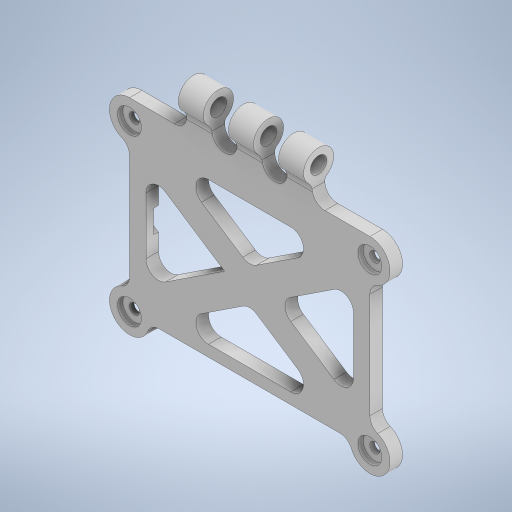
# Autodesk Inventor part: polycase_bracket
Saved by Autodesk Inventor 2024 (Build 280153000, 153)
## iProperties
Created: 2024-04-12
Part Number: polycase_bracket
Material: Generic
Document SubType Name: Modeling
Designer: Jacob
Density: 1 g/cm^3
Appearance: Default
Author: Jacob
## iProperties of the stored document polycase_bracket_3DPrint.ipt
Created: 2024-04-15
Part Number: polycase_bracket_3DPrint
Material: Generic
Document SubType Name: Modeling
Designer: Jacob
Density: 1 g/cm^3
Appearance: Default
Author: Jacob
Autodesk Inventor part; units mm, degrees
ref_plane "YZ Plane" through (0, 0, 0) normal (1, 0, 0) x (0, 1, 0)
ref_plane "XZ Plane" through (0, 0, 0) normal (0, 1, 0) x (-1, 0, 0)
ref_plane "XY Plane" through (0, 0, 0) normal (0, 0, 1) x (1, 0, 0)
sketch "Sketch1" plane through (0, 0, 0) normal (0, 0, 1) x (1, 0, 0)
  line L0 (48, -33) -> (-48, -33)
  line L1 (-48, -33) -> (-48, 33)
  line L2 (-48, 33) -> (48, 33)
  line L3 (48, 33) -> (48, -33)
  line L4 (48, -33) -> (-48, 33) construction
  line L5 (-48, -33) -> (48, 33) construction
  circle A0 centre (-48, 33) radius 1.727
  circle A1 centre (48, 33) radius 1.727
  circle A2 centre (-48, -33) radius 1.727
  circle A3 centre (48, -33) radius 1.727
  circle A4 centre (-48, 33) radius 8
  circle A5 centre (48, 33) radius 8
  circle A6 centre (48, -33) radius 8
  circle A7 centre (-48, -33) radius 8
  line L6 (41.4077, -28.4678) -> (-41.4077, -28.4678)
  line L7 (-41.4077, -28.4678) -> (-41.4077, 28.4678)
  line L8 (-41.4077, 28.4678) -> (41.4077, 28.4678)
  line L9 (41.4077, 28.4678) -> (41.4077, -28.4678)
  line L10 (41.4077, -28.4678) -> (-41.4077, 28.4678) construction
  line L11 (-41.4077, -28.4678) -> (41.4077, 28.4678) construction
  line L12 (-40, -33) -> (48, 25)
  line L13 (40, 33) -> (-48, -25)
  line L14 (-40, 33) -> (48, -25)
  line L15 (40, -33) -> (-48, 25)
  line L16 (56, 33) -> (56, -33)
  line L17 (-48, 41) -> (48, 41)
  line L18 (-56, 33) -> (-56, -33)
  line L19 (-48, -41) -> (48, -41)
  point P0 (0, 0)
  point P1 (-33.1235, -28.4678)
  point P2 (0, -6.6364)
  point P3 (33.1235, -28.4678)
  point P4 (41.4077, 20.6551)
  point P5 (41.4077, -20.6551)
  point P6 (10.069, 0)
  point P7 (33.1235, 28.4678)
  point P8 (0, 6.6364)
  point P9 (-33.1235, 28.4678)
  point P10 (-41.4077, -20.6551)
  point P11 (-41.4077, 20.6551)
  point P12 (-10.069, 0)
  dimension "d0" = 96
  dimension "d1" = 66
  dimension "d2" = 3.454
  dimension "d3" = 3.454
  dimension "d4" = 3.454
  dimension "d5" = 3.454
  dimension "d6" = 16
  dimension "d7" = 16
  dimension "d8" = 16
  dimension "d9" = 16
  constraints: 40 end point, 17 point on circle, 8 centre point, 8 coincident, 6 point on line, 4 midpoint, 4 parallel, 4 perpendicular, 2 horizontal, 2 tangent
  measures "d0" distance of L1.end L2.end
  measures "d1" distance of L0.end L1.end
  measures "d2" diameter of A0
  measures "d3" diameter of A1
  measures "d4" diameter of A2
  measures "d5" diameter of A3
  measures "d6" diameter of A4
  measures "d7" diameter of A5
  measures "d8" diameter of A6
  measures "d9" diameter of A7
extrude "Extrusion1" add sketch "Sketch1" along normal blind 5 contours A6 L3 A3 L0 | L15 L6 A6 | L0 A3 L3 A6 | L0 L12 L6 L15 | A7 L1 A2 L0 | L0 A2 L1 A7 | A7 L6 L12 | L9 L14 A6 | L6 L15 L12 L14 L9 | L7 L13 L15 L12 L6 | A7 L13 L7 | L14 L9 L12 L3 | L15 L13 L14 L12 | L1 L15 L7 L13 | A5 L2 A1 L3 | L12 L9 A5 | L3 A1 L2 A5 | L12 L14 L13 L8 L9 | L15 L7 L8 L14 L13 | A4 L2 A0 L1 | L1 A0 L2 A4 | A4 L7 L15 | L8 L13 A5 | A4 L14 L8 | L13 L8 L14 L2
fillet "Fillet1" radius 5 19 edges at (-40, 33, 2.5) (-48, 25, 2.5) (-33.1235, 28.4678, 2.5) (-41.4077, 20.6551, 2.5) (0, 6.6364, 2.5) (10.069, 0, 2.5) (33.1235, 28.4678, 2.5) (41.4077, 20.6551, 2.5) (40, 33, 2.5) (48, 25, 2.5) (41.4077, -20.6551, 2.5) (33.1235, -28.4678, 2.5) (0, -6.6364, 2.5) (-33.1235, -28.4678, 2.5) (-41.4077, -20.6551, 2.5) (48, -25, 2.5) (40, -33, 2.5) (-40, -33, 2.5) (-48, -25, 2.5)
sketch "Sketch2" plane through (0, 0, 0) normal (0, 0, -1) x (-1, 0, 0)
  circle A0 centre (-48, 33) radius 1.727 projected
  circle A1 centre (-48, 33) radius 2
  circle A2 centre (48, 33) radius 1.727 projected
  circle A3 centre (48, 33) radius 2
  circle A4 centre (48, -33) radius 1.727 projected
  circle A5 centre (48, -33) radius 2
  circle A6 centre (-48, -33) radius 1.727 projected
  circle A7 centre (-48, -33) radius 2
  circle A8 centre (-48, 33) radius 4.75
  circle A9 centre (48, 33) radius 1.727 projected
  circle A10 centre (48, 33) radius 4.75
  circle A11 centre (48, -33) radius 4.75
  circle A12 centre (-48, -33) radius 4.75
  point P0 (0, 0)
  dimension "d13" = 4
  dimension "d14" = 4
  dimension "d15" = 4
  dimension "d16" = 4
  dimension "d17" = 9.5
  dimension "d18" = 9.5
  dimension "d19" = 9.5
  dimension "d20" = 9.5
  constraints: 8 centre point, 8 coincident
  measures "d13" diameter of A1
  measures "d14" diameter of A3
  measures "d15" diameter of A5
  measures "d16" diameter of A7
  measures "d17" diameter of A8
  measures "d18" diameter of A10
  measures "d19" diameter of A11
  measures "d20" diameter of A12
extrude "Extrusion2" cut sketch "Sketch2" against normal blind 5 contours A0 | A1 | A2 | A3 | A4 | A5 | A6 | A7
extrude "Extrusion3" cut sketch "Sketch2" against normal blind 1.2 contours A8 | A10 | A11 | A12
sketch "Sketch3" plane through (-36, 33, 0) normal (0, 1, 0) x (1, 0, 0)
  line L0 (86, -5) -> (82, -5) projected
  line L1 (-14, 5) -> (86, 5)
  line L2 (86, 5) -> (86, -5)
  line L3 (86, -5) -> (-14, -5)
  line L4 (-14, -5) -> (-14, 5)
  line L5 (-14, 5) -> (86, -5) construction
  line L6 (86, 5) -> (-14, -5) construction
  line L7 (76.6154, 0) -> (92, 0) projected
  line L8 (-14, -5) -> (86, -5)
  line L9 (86, -5) -> (86, 0)
  line L10 (86, 0) -> (-14, 0)
  line L11 (-14, 0) -> (-14, -5)
  line L12 (-4.6154, -5) -> (0, -5) projected
  line L13 (76.6154, 0) -> (-4.6154, 0)
  line L14 (-4.6154, 0) -> (-4.6154, -5)
  line L15 (-4.6154, -5) -> (76.6154, -5)
  line L16 (76.6154, -5) -> (76.6154, 0)
  line L17 (11, 5) -> (61, 5)
  line L18 (61, 5) -> (61, -5)
  line L19 (61, -5) -> (11, -5)
  line L20 (11, -5) -> (11, 5)
  line L21 (11, 5) -> (61, -5) construction
  line L22 (61, 5) -> (11, -5) construction
  line L23 (0, 0) -> (72, 0) projected
  line L24 (61, -5) -> (11, -5)
  line L25 (11, -5) -> (11, 0)
  line L26 (11, 0) -> (61, 0)
  line L27 (61, 0) -> (61, -5)
  line L28 (11, -5) -> (21, -5)
  line L29 (21, -5) -> (21, 0)
  line L30 (21, 0) -> (11, 0)
  line L31 (11, 0) -> (11, -5)
  line L32 (61, -5) -> (51, -5)
  line L33 (51, -5) -> (51, 0)
  line L34 (51, 0) -> (61, 0)
  line L35 (61, 0) -> (61, -5)
  line L36 (31, 5) -> (41, 5)
  line L37 (41, 5) -> (41, -5)
  line L38 (41, -5) -> (31, -5)
  line L39 (31, -5) -> (31, 5)
  line L40 (31, 5) -> (41, -5) construction
  line L41 (41, 5) -> (31, -5) construction
  line L42 (31, 0) -> (41, 0)
  point P0 (36, 0)
  point P1 (87.0769, 0)
  dimension "d25" = 50
  dimension "d26" = 10
  dimension "d27" = 10
  dimension "d28" = 10
  constraints: 78 end point, 16 parallel, 10 midpoint, 8 horizontal, 8 perpendicular, 6 point on line
  measures "d25" distance of L18.end L19.end
  measures "d26" distance of L30.end L29.end
  measures "d27" distance of L33.end L34.end
  measures "d28" distance of L37.end L38.end
extrude "Extrusion4" add sketch "Sketch3" along normal blind 20 contours L3 L33 L10 L18 | L3 L39 L10 L37 | L3 L20 L10 L29
sketch "Sketch4" plane through (25, 33, 5) normal (1, 0, 0) x (0, 0, -1)
  line L0 (5, 0) -> (5, 20) projected
  line L1 (5, 10) -> (0, 10)
  line L2 (0, 0) -> (0, 20) projected
  line L3 (0, 20) -> (5, 20) projected
  line L4 (2.5, 20) -> (2.5, 15)
  circle A0 centre (2.5, 15) radius 3.25
  circle A1 centre (2.5, 15) radius 6
  point P0 (5, -33)
  point P1 (5, 9.5456)
  point P2 (0, 9.5456)
  point P3 (0, 12.9233)
  point P4 (0, 17.0767)
  point P5 (5, 17.0767)
  point P6 (5, 12.9233)
  dimension "d31" = 5
  dimension "d32" = 6.5
  dimension "d33" = 12
  constraints: 4 end point, 3 midpoint, 2 centre point, 2 coincident, 1 vertical
  measures "d31" distance of L4.start L4.end
  measures "d32" diameter of A0
  measures "d33" diameter of A1
extrude "Extrusion5" add sketch "Sketch4" against normal up to surface (10 mm away) contours L0 A0 L3 L2 A1
extrude "Extrusion6" cut sketch "Sketch4" against normal blind 10 contours A0 L2 L0 | L0 A0 | A0 L2
sketch "Sketch5" plane through (5, 33, 5) normal (1, 0, 0) x (0, 0, -1)
  circle A0 centre (2.5, 15) radius 3.25 projected
  arc A1 (5, 9.5456) -> (0, 9.5456) centre (2.5, 15) ccw projected
  circle A2 centre (2.5, 15) radius 6
  point P0 (5, -33)
  point P1 (0, 9.5456)
  point P2 (5, 9.5456)
  constraints: 1 centre point, 1 coincident, 1 concentric
extrude "Extrusion7" add sketch "Sketch5" against normal up to surface (10 mm away)
extrude "Extrusion8" cut sketch "Sketch5" against normal blind 10 contours A0
sketch "Sketch6" plane through (-15, 33, 5) normal (1, 0, 0) x (0, 0, -1)
  circle A0 centre (2.5, 15) radius 3.25 projected
  circle A1 centre (2.5, 15) radius 3.25
  circle A2 centre (2.5, 15) radius 6
  point P0 (5, -33)
  constraints: 2 centre point, 2 coincident
extrude "Extrusion9" add sketch "Sketch6" against normal up to surface (10 mm away)
extrude "Extrusion10" cut sketch "Sketch6" against normal up to surface (10 mm away) contours A0
fillet "Fillet2" radius 2 3 edges at (20, 42.5456, 0) (0, 42.5456, 0) (-20, 42.5456, 0)
fillet "Fillet3" radius 5 9 edges at (-20, 42.5456, 5) (0, 42.5456, 5) (20, 42.5456, 5) (15, 33, 2.5) (5, 33, 2.5) (-5, 33, 2.5) (-15, 33, 2.5) (25, 33, 2.5) (-25, 33, 2.5)
sketch "Sketch8" plane through (0, 0, 5) normal (0, 0, 1) x (1, 0, 0)
  circle A0 centre (-48, 33) radius 2 projected
  circle A1 centre (-48, 33) radius 4.75
  circle A2 centre (48, 33) radius 2 projected
  circle A3 centre (48, 33) radius 4.75
  circle A4 centre (48, -33) radius 2 projected
  circle A5 centre (48, -33) radius 4.75
  circle A6 centre (-48, -33) radius 2 projected
  circle A7 centre (-48, -33) radius 4.75
  point P0 (0, 0)
  dimension "d50" = 9.5
  dimension "d51" = 9.5
  dimension "d52" = 9.5
  dimension "d53" = 9.5
  constraints: 4 centre point, 4 coincident
  measures "d50" diameter of A1
  measures "d51" diameter of A3
  measures "d52" diameter of A5
  measures "d53" diameter of A7
extrude "Extrusion12" cut sketch "Sketch8" against normal blind 2 contours A0 | A1 | A2 | A3 | A4 | A5 | A6 | A7
sketch "Sketch9" plane through (0, 0, 0) normal (0, 0, -1) x (-1, 0, 0)
  line L0 (55.3401, -40.9684) -> (-55.3401, -40.9684) projected
  spline S0 degree 3 poles (-55.3401, -40.9684) (-55.4056, -40.9684) (-55.471, -40.9554) (-55.5315, -40.9303) (-55.5919, -40.9053) (-55.6474, -40.8682) (-55.6937, -40.822) (-55.7399, -40.7757) (-55.777, -40.7202) (-55.802, -40.6598) (-55.8271, -40.5993) (-55.8401, -40.5339) (-55.8401, -40.4684) knots 5.497939 5.497939 5.497939 5.497939 5.890562 5.890562 5.890562 6.283185 6.283185 6.283185 6.675808 6.675808 6.675808 7.068431 7.068431 7.068431 7.068431 projected
  line L1 (-55.8401, -40.4684) -> (-55.8401, 40.4684) projected
  spline S1 degree 3 poles (-55.8401, 40.4684) (-55.8401, 40.5339) (-55.8271, 40.5993) (-55.802, 40.6598) (-55.777, 40.7202) (-55.7399, 40.7757) (-55.6937, 40.822) (-55.6474, 40.8682) (-55.5919, 40.9053) (-55.5315, 40.9303) (-55.471, 40.9554) (-55.4056, 40.9684) (-55.3401, 40.9684) knots 5.497939 5.497939 5.497939 5.497939 5.890562 5.890562 5.890562 6.283185 6.283185 6.283185 6.675808 6.675808 6.675808 7.068431 7.068431 7.068431 7.068431 projected
  line L2 (-55.3401, 40.9684) -> (55.3401, 40.9684) projected
  spline S2 degree 3 poles (55.3401, 40.9684) (55.4056, 40.9684) (55.471, 40.9554) (55.5315, 40.9303) (55.5919, 40.9053) (55.6474, 40.8682) (55.6937, 40.822) (55.7399, 40.7757) (55.777, 40.7202) (55.802, 40.6598) (55.8271, 40.5993) (55.8401, 40.5339) (55.8401, 40.4684) knots 5.497939 5.497939 5.497939 5.497939 5.890562 5.890562 5.890562 6.283185 6.283185 6.283185 6.675808 6.675808 6.675808 7.068431 7.068431 7.068431 7.068431 projected
  line L3 (55.8401, 40.4684) -> (55.8401, -40.4684) projected
  spline S3 degree 3 poles (55.8401, -40.4684) (55.8401, -40.5339) (55.8271, -40.5993) (55.802, -40.6598) (55.777, -40.7202) (55.7399, -40.7757) (55.6937, -40.822) (55.6474, -40.8682) (55.5919, -40.9053) (55.5315, -40.9303) (55.471, -40.9554) (55.4056, -40.9684) (55.3401, -40.9684) knots 5.497939 5.497939 5.497939 5.497939 5.890562 5.890562 5.890562 6.283185 6.283185 6.283185 6.675808 6.675808 6.675808 7.068431 7.068431 7.068431 7.068431 projected
  line L4 (29.8976, -1.9965) -> (31.7769, -2.8744) projected
  line L5 (29.8976, -2.0069) -> (29.8976, -1.9965) projected
  line L6 (28.292, -2.9083) -> (29.8976, -2.0069) projected
  line L7 (28.292, -3.3844) -> (28.292, -2.9083) projected
  line L8 (29.8556, -2.4469) -> (28.292, -3.3844) projected
  line L9 (31.7769, -3.3844) -> (29.8556, -2.4469) projected
  line L10 (31.7769, -2.8744) -> (31.7769, -3.3844) projected
  line L11 (31.7769, 5.9658) -> (31.7769, 4.5059) projected
  line L12 (28.292, 5.9658) -> (31.7769, 5.9658) projected
  line L13 (28.292, 4.553) -> (28.292, 5.9658) projected
  line L14 (28.6687, 4.553) -> (28.292, 4.553) projected
  line L15 (28.6687, 5.542) -> (28.6687, 4.553) projected
  line L16 (29.799, 5.542) -> (28.6687, 5.542) projected
  line L17 (29.799, 4.6001) -> (29.799, 5.542) projected
  line L18 (30.1757, 4.6001) -> (29.799, 4.6001) projected
  line L19 (30.1757, 5.542) -> (30.1757, 4.6001) projected
  line L20 (31.4001, 5.542) -> (30.1757, 5.542) projected
  line L21 (31.4001, 4.5059) -> (31.4001, 5.542) projected
  line L22 (31.7769, 4.5059) -> (31.4001, 4.5059) projected
  line L23 (31.7769, 1.5391) -> (28.8115, 1.5391) projected
  line L24 (31.7769, 1.9629) -> (31.7769, 1.5391) projected
  line L25 (28.292, 1.9629) -> (31.7769, 1.9629) projected
  line L26 (28.292, 1.269) -> (28.292, 1.9629) projected
  line L27 (31.2846, 0.503) -> (28.292, 1.269) projected
  line L28 (28.292, 0.503) -> (31.2846, 0.503) projected
  line L29 (28.292, 0.0792) -> (28.292, 0.503) projected
  line L30 (31.7769, 0.0792) -> (28.292, 0.0792) projected
  line L31 (31.7769, 0.7797) -> (31.7769, 0.0792) projected
  line L32 (28.8115, 1.5391) -> (31.7769, 0.7797) projected
  line L33 (31.7769, -8.3976) -> (31.7769, -9.8574) projected
  line L34 (28.292, -8.3976) -> (31.7769, -8.3976) projected
  line L35 (28.292, -9.8104) -> (28.292, -8.3976) projected
  line L36 (28.6687, -9.8104) -> (28.292, -9.8104) projected
  line L37 (28.6687, -8.8214) -> (28.6687, -9.8104) projected
  line L38 (29.799, -8.8214) -> (28.6687, -8.8214) projected
  line L39 (29.799, -9.7633) -> (29.799, -8.8214) projected
  line L40 (30.1757, -9.7633) -> (29.799, -9.7633) projected
  line L41 (30.1757, -8.8214) -> (30.1757, -9.7633) projected
  line L42 (31.4001, -8.8214) -> (30.1757, -8.8214) projected
  line L43 (31.4001, -9.8574) -> (31.4001, -8.8214) projected
  line L44 (31.7769, -9.8574) -> (31.4001, -9.8574) projected
  line L45 (31.7769, -10.2342) -> (31.7769, -10.6536) projected
  line L46 (28.292, -10.9553) -> (31.7769, -10.2342) projected
  line L47 (28.292, -11.5204) -> (28.292, -10.9553) projected
  line L48 (31.7769, -12.2415) -> (28.292, -11.5204) projected
  line L49 (31.7769, -11.7838) -> (31.7769, -12.2415) projected
  line L50 (30.9763, -11.6367) -> (31.7769, -11.7838) projected
  line L51 (30.9763, -10.803) -> (30.9763, -11.6367) projected
  line L52 (31.7769, -10.6536) -> (30.9763, -10.803) projected
  circle A0 centre (39.4888, 19.5371) radius 4.127 projected
  line L53 (31.7769, -6.1371) -> (31.7769, -6.5609) projected
  line L54 (28.292, -6.1371) -> (31.7769, -6.1371) projected
  line L55 (28.292, -7.1231) -> (28.292, -6.1371) projected
  spline S4 degree 3 poles (29.1536, -7.8795) (29.0848, -7.8799) (28.985, -7.874) (28.8571, -7.8556) (28.772, -7.8348) (28.6936, -7.8094) (28.6229, -7.7765) (28.5583, -7.7396) (28.5018, -7.6954) (28.4517, -7.6458) (28.4091, -7.5893) (28.3725, -7.5269) (28.3436, -7.4579) (28.3194, -7.3833) (28.2983, -7.2712) (28.2908, -7.1835) (28.292, -7.1231) knots 0 0 0 0 0.156529 0.227063 0.293634 0.355378 0.41429 0.470549 0.524222 0.577081 0.630415 0.684665 0.741142 0.800246 0.862827 1 1 1 1 projected
  spline S5 degree 3 poles (29.8026, -7.6676) (29.7671, -7.7045) (29.7032, -7.7511) (29.6071, -7.7992) (29.5249, -7.8284) (29.4354, -7.8521) (29.3373, -7.8676) (29.2426, -7.877) (29.1804, -7.8793) (29.1536, -7.8795) knots 0.046127 0.046127 0.046127 0.046127 0.254948 0.367127 0.484568 0.611118 0.745389 0.890554 1 1 1 1 projected
  spline S6 degree 3 poles (29.991, -7.2614) (29.9755, -7.3413) (29.9387, -7.4908) (29.8517, -7.6179) (29.8026, -7.6676) knots 0 0 0 0 0.539837 1 1 1 1 projected
  spline S7 degree 3 poles (30.1404, -7.6588) (30.1182, -7.6394) (30.0896, -7.6041) (30.0588, -7.5498) (30.0383, -7.5028) (30.0216, -7.4499) (30.0022, -7.3696) (29.995, -7.3055) (29.991, -7.2614) knots 0 0 0 0 0.202398 0.311642 0.429962 0.556371 0.693993 1 1 1 1 projected
  spline S8 degree 3 poles (30.729, -7.7971) (30.6623, -7.7954) (30.5661, -7.7923) (30.4447, -7.7752) (30.3661, -7.7616) (30.2971, -7.7412) (30.2194, -7.7131) (30.1687, -7.6826) (30.1404, -7.6588) knots 0 0 0 0 0.326051 0.468546 0.597628 0.71466 0.819562 1 1 1 1 projected
  spline S9 degree 3 poles (31.2603, -7.8236) (31.1805, -7.8163) (31.0036, -7.8023) (30.8262, -7.7996) (30.729, -7.7971) knots 0 0 0 0 0.452087 1 1 1 1 projected
  line L56 (31.3427, -7.8324) -> (31.2603, -7.8236) projected
  spline S10 degree 3 poles (31.7769, -7.9082) (31.7111, -7.8908) (31.5673, -7.8594) (31.4211, -7.8423) (31.3427, -7.8324) knots 0 0 0 0 0.46278 1 1 1 1 projected
  line L57 (31.7769, -7.4572) -> (31.7769, -7.9082) projected
  spline S11 degree 3 poles (31.3751, -7.3924) (31.4247, -7.3968) (31.4906, -7.4065) (31.5761, -7.4198) (31.6604, -7.4368) (31.7289, -7.4466) (31.7769, -7.4572) knots 0 0 0 0 0.366384 0.490892 0.638013 1 1 1 1 projected
  line L58 (31.3, -7.3858) -> (31.3751, -7.3924) projected
  spline S12 degree 3 poles (30.8107, -7.3615) (30.8964, -7.3628) (31.0597, -7.3674) (31.2226, -7.3793) (31.3, -7.3858) knots 0 0 0 0 0.524335 1 1 1 1 projected
  spline S13 degree 3 poles (30.1757, -6.884) (30.1759, -6.923) (30.1789, -6.9803) (30.1952, -7.0525) (30.2113, -7.1003) (30.2313, -7.144) (30.2561, -7.1833) (30.2871, -7.217) (30.321, -7.2483) (30.3618, -7.2737) (30.4075, -7.2968) (30.4598, -7.3156) (30.518, -7.332) (30.5826, -7.3438) (30.6805, -7.3576) (30.7575, -7.3602) (30.8107, -7.3615) knots 0 0 0 0 0.128242 0.186728 0.241872 0.293283 0.343884 0.393401 0.442919 0.49463 0.550334 0.61034 0.67624 0.748264 0.825316 1 1 1 1 projected
  line L59 (30.1757, -6.5609) -> (30.1757, -6.884) projected
  line L60 (31.7769, -6.5609) -> (30.1757, -6.5609) projected
  spline S14 degree 3 poles (31.824, -4.6772) (31.8244, -4.7511) (31.817, -4.8582) (31.7939, -4.9948) (31.7679, -5.0848) (31.7354, -5.1669) (31.696, -5.2409) (31.6483, -5.3064) (31.5932, -5.3639) (31.5296, -5.4137) (31.4576, -5.4565) (31.3768, -5.4925) (31.287, -5.5219) (31.1882, -5.5444) (31.0389, -5.5662) (30.9218, -5.573) (30.8409, -5.572) knots 0 0 0 0 0.143629 0.208619 0.269211 0.32577 0.380025 0.431972 0.482955 0.534624 0.588579 0.645631 0.706471 0.772131 0.842618 1 1 1 1 projected
  spline S15 degree 3 poles (30.6452, -3.7825) (30.7484, -3.783) (30.8972, -3.7862) (31.0859, -3.8082) (31.2085, -3.828) (31.3181, -3.8549) (31.4147, -3.8879) (31.4985, -3.9265) (31.5705, -3.9721) (31.6317, -4.0264) (31.6835, -4.0905) (31.7269, -4.1644) (31.7635, -4.2474) (31.79, -4.3411) (31.8172, -4.4846) (31.8248, -4.5985) (31.824, -4.6772) knots 0 0 0 0 0.17898 0.257216 0.328718 0.393925 0.452355 0.505367 0.553318 0.599348 0.646446 0.695395 0.747319 0.803095 0.863654 1 1 1 1 projected
  line L61 (29.3567, -3.7825) -> (30.6452, -3.7825) projected
  spline S16 degree 3 poles (28.2449, -4.6772) (28.2458, -4.6035) (28.2513, -4.4957) (28.2796, -4.3596) (28.308, -4.2691) (28.3453, -4.1872) (28.3899, -4.1131) (28.4436, -4.0476) (28.5056, -3.99) (28.5772, -3.9406) (28.6584, -3.8975) (28.7501, -3.8618) (28.8519, -3.8327) (28.9636, -3.81) (29.1326, -3.7882) (29.2651, -3.7816) (29.3567, -3.7825) knots 0 0 0 0 0.134219 0.195262 0.252375 0.306254 0.358487 0.409187 0.459672 0.511874 0.56693 0.626384 0.690452 0.759189 0.833415 1 1 1 1 projected
  spline S17 degree 3 poles (29.3744, -5.572) (29.2801, -5.5722) (29.1436, -5.5671) (28.9697, -5.5453) (28.8552, -5.5223) (28.7513, -5.4944) (28.6583, -5.4589) (28.5763, -5.4171) (28.504, -5.3689) (28.4421, -5.3122) (28.389, -5.2469) (28.3444, -5.173) (28.3071, -5.0906) (28.2798, -4.9991) (28.2509, -4.8615) (28.246, -4.7521) (28.2449, -4.6772) knots 0 0 0 0 0.169293 0.244767 0.314365 0.378777 0.437733 0.492673 0.543718 0.593269 0.642711 0.694286 0.747888 0.80457 0.865275 1 1 1 1 projected
  line L62 (30.8409, -5.572) -> (29.3744, -5.572) projected
  line L63 (31.7769, -1.9929) -> (28.292, -1.9929) projected
  line L64 (31.7769, -1.5691) -> (31.7769, -1.9929) projected
  line L65 (28.292, -1.5691) -> (31.7769, -1.5691) projected
  line L66 (28.292, -1.9929) -> (28.292, -1.5691) projected
  line L67 (31.7769, 2.9989) -> (31.7769, 2.5751) projected
  line L68 (28.292, 2.9989) -> (31.7769, 2.9989) projected
  line L69 (28.292, 2.5751) -> (28.292, 2.9989) projected
  line L70 (31.7769, 2.5751) -> (28.292, 2.5751) projected
  line L71 (31.7769, 8.2733) -> (31.7769, 7.2704) projected
  line L72 (28.292, 8.2733) -> (31.7769, 8.2733) projected
  line L73 (28.292, 7.5088) -> (28.292, 8.2733) projected
  spline S18 degree 3 poles (29.3221, 6.4838) (29.2374, 6.4842) (29.1142, 6.4892) (28.9577, 6.5158) (28.8539, 6.5417) (28.7595, 6.5759) (28.6742, 6.6165) (28.5992, 6.6666) (28.5327, 6.7235) (28.475, 6.7897) (28.4258, 6.8651) (28.3849, 6.95) (28.3497, 7.0433) (28.3238, 7.1466) (28.2991, 7.3023) (28.2912, 7.4244) (28.292, 7.5088) knots 0 0 0 0 0.150899 0.218633 0.282146 0.341098 0.396924 0.449822 0.501186 0.55222 0.605482 0.660916 0.71961 0.7827 0.849931 1 1 1 1 projected
  line L74 (30.6805, 6.4838) -> (29.3221, 6.4838) projected
  spline S19 degree 3 poles (31.7769, 7.2704) (31.7779, 7.2053) (31.7695, 7.1108) (31.7431, 6.991) (31.714, 6.9119) (31.6778, 6.8396) (31.6338, 6.774) (31.5797, 6.7173) (31.5187, 6.6661) (31.4477, 6.6228) (31.3676, 6.5852) (31.2775, 6.5538) (31.1774, 6.5285) (31.0677, 6.5076) (30.901, 6.4894) (30.7706, 6.4835) (30.6805, 6.4838) knots 0 0 0 0 0.125725 0.182644 0.23663 0.288145 0.338633 0.388605 0.439102 0.492114 0.54873 0.610049 0.67616 0.748027 0.825817 1 1 1 1 projected
  line L75 (31.7769, 10.7693) -> (31.7769, 10.3499) projected
  line L76 (28.292, 10.0482) -> (31.7769, 10.7693) projected
  line L77 (28.292, 9.483) -> (28.292, 10.0482) projected
  line L78 (31.7769, 8.7619) -> (28.292, 9.483) projected
  line L79 (31.7769, 9.2196) -> (31.7769, 8.7619) projected
  line L80 (30.9763, 9.3668) -> (31.7769, 9.2196) projected
  line L81 (30.9763, 10.2005) -> (30.9763, 9.3668) projected
  line L82 (31.7769, 10.3499) -> (30.9763, 10.2005) projected
  line L83 (31.7769, 13.3594) -> (28.7521, 13.3594) projected
  line L84 (31.7769, 13.7832) -> (31.7769, 13.3594) projected
  line L85 (28.292, 13.7832) -> (31.7769, 13.7832) projected
  line L86 (28.292, 13.0577) -> (28.292, 13.7832) projected
  line L87 (31.0868, 12.5018) -> (28.292, 13.0577) projected
  line L88 (28.292, 11.9657) -> (31.0868, 12.5018) projected
  line L89 (28.292, 11.2402) -> (28.292, 11.9657) projected
  line L90 (31.7769, 11.2402) -> (28.292, 11.2402) projected
  line L91 (31.7769, 11.664) -> (31.7769, 11.2402) projected
  line L92 (28.7582, 11.664) -> (31.7769, 11.664) projected
  line L93 (31.7769, 12.2939) -> (28.7582, 11.664) projected
  line L94 (31.7769, 12.7266) -> (31.7769, 12.2939) projected
  line L95 (28.7521, 13.3594) -> (31.7769, 12.7266) projected
  line L96 (18.2158, -13.97) -> (18.2158, 13.97) projected
  line L97 (27.2328, -13.97) -> (18.2158, -13.97) projected
  line L98 (27.2328, 13.97) -> (27.2328, -13.97) projected
  line L99 (18.2158, 13.97) -> (27.2328, 13.97) projected
  circle A1 centre (-40, 0) radius 4.8 projected
  circle A2 centre (48, -33) radius 4.699 projected
  circle A3 centre (-48, 33) radius 4.699 projected
  circle A4 centre (0, 0) radius 8.001 projected
  circle A5 centre (-48, -33) radius 4.699 projected
  circle A6 centre (48, 33) radius 4.699 projected
  circle A7 centre (40, 0) radius 4.8 projected
  point P0 (0, 0)
extrude "Extrusion13" cut sketch "Sketch9" against normal blind 2 contours A1 | A7
sketch "Sketch18" plane through (0, 0, 0) normal (0, 0, -1) x (-1, 0, 0)
  line L0 (25, 38) -> (25, 39.9533) projected
  line L1 (-25, 38) -> (-25, 39.9533) projected
  line L2 (25, 38) -> (-25, 38)
  line L3 (-25, 38) -> (25, 38)
  line L4 (25, 38) -> (25, 67.3319)
  line L5 (25, 67.3319) -> (-25, 67.3319)
  line L6 (-25, 67.3319) -> (-25, 38)
  point P0 (0, 0)
  constraints: 10 end point, 2 horizontal, 2 parallel, 1 perpendicular
split body "Split2" sketch "Sketch18" result two bodies curves L4 L5 L6 L3 first body at (-21.6667, 44.2983, 6.5679) (1.6667, 51.0042, 7.107) (18.3333, 44.6451, 6.8583)
move or copy body "Move Body1" bodies to move or copy 2 copy no translate (0, 5, 0)
sketch "Sketch19" plane through (-25, 38, 0) normal (0, 1, 0) x (1, 0, 0)
  line L0 (0, 0) -> (10, 0) projected
  line L1 (0, -5) -> (0, 0) projected
  line L2 (10, -5) -> (0, -5) projected
  line L3 (10, 0) -> (10, -5) projected
  line L4 (30, 0) -> (30, -5) projected
  line L5 (20, 0) -> (30, 0) projected
  line L6 (20, -5) -> (20, 0) projected
  line L7 (30, -5) -> (20, -5) projected
  line L8 (40, 0) -> (50, 0) projected
  line L9 (40, -5) -> (40, 0) projected
  line L10 (50, -5) -> (40, -5) projected
  line L11 (50, 0) -> (50, -5) projected
  point P0 (25, 0)
extrude "Extrusion21" add sketch "Sketch19" along normal up to surface (5 mm away) bodies 3
combine bodies "Combine1" operation type add bodies to combine 3 2
sketch "Sketch20" plane through (36, -33, 0) normal (0, 0, -1) x (-1, 0, 0)
  arc A0 (87.0769, 58.6154) -> (76.6154, 69.0769) centre (84, 66) ccw projected
  circle A1 centre (-12, 66) radius 2 projected
  line L0 (84, 74) -> (-12, 74)
  line L1 (-12, 74) -> (-12, 66)
  line L2 (-12, 66) -> (84, 66)
  line L3 (84, 66) -> (84, 74)
  circle A2 centre (-12, 66) radius 4.75
  circle A3 centre (84, 66) radius 4.75 projected
  circle A4 centre (84, 66) radius 4.75
  point P0 (36, 33)
  point P1 (79.25, 66)
  point P2 (84, 70.75)
  point P3 (-12, 70.75)
  point P4 (-7.25, 66)
  constraints: 8 end point, 2 centre point, 2 coincident, 2 parallel, 1 horizontal, 1 perpendicular, 1 point on circle
extrude "Extrusion22" add sketch "Sketch20" against normal up to surface (5 mm away) contours A2 L1 L0 L3 A3 L2 bodies 3
fillet "Fillet5" radius 5 6 edges at (15, 41, 2.5) (5, 41, 2.5) (-5, 41, 2.5) (-15, 41, 2.5) (-25, 41, 2.5) (25, 41, 2.5)
body "Solid3"
